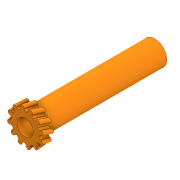
# Autodesk Inventor part: 6th Axis Drive Gear
Saved by Autodesk Inventor 2020 (Build 240168000, 168)
## iProperties
Created: 2021-06-26
Part Number: 6th Axis Drive Gear
Material: Generic
Document SubType Name: Modeling
Designer: Coy
Density: 1 g/cm^3
Appearance: Orange
Author: Coy
Autodesk Inventor part; units mm, degrees
ref_plane "YZ Plane" through (0, 0, 0) normal (1, 0, 0) x (0, 1, 0)
ref_plane "XZ Plane" through (0, 0, 0) normal (0, 1, 0) x (-1, 0, 0)
ref_plane "XY Plane" through (0, 0, 0) normal (0, 0, 1) x (1, 0, 0)
sketch "Sketch1" plane through (0, 0, 0) normal (0, 0, 1) x (1, 0, 0)
  circle A0 centre (0, 0) radius 6
  circle A1 centre (0, 0) radius 4
  dimension "d0" = 12
  dimension "d1" = 8
  constraints: 2 centre point, 2 coincident
  measures "d0" diameter of A0
  measures "d1" diameter of A1
extrude "Extrusion1" add sketch "Sketch1" along normal blind 64
ref_plane "Work Plane1" through (0, 0, 59) normal (0, 0, 1) x (1, 0, 0)
sketch "Sketch3" plane through (0, 0, 59) normal (0, 0, 1) x (1, 0, 0)
  circle A0 centre (0, 0) radius 9 construction
  line L0 (0, 0) -> (0, 12.6583) construction
  arc A1 (0.9922, 7.875) -> (-0.9922, 7.875) centre (0, 8) ccw
  line L1 (0.967, 7.675) -> (0.9922, 7.875)
  line L2 (-0.967, 7.675) -> (-0.9922, 7.875)
  arc A2 (-1.7079, 6.582) -> (-0.967, 7.675) centre (-1.9591, 7.55) ccw
  arc A3 (0.967, 7.675) -> (1.7079, 6.582) centre (1.9591, 7.55) ccw
  arc A4 (-4.7701, 4.8462) -> (-4.6749, 6.1632) centre (-5.4716, 5.5589) ccw
  line L3 (-4.6749, 6.1632) -> (-4.7967, 6.3239)
  arc A5 (-3.0783, 7.316) -> (-4.7967, 6.3239) centre (-4, 6.9282) ccw
  line L4 (-3.0001, 7.1302) -> (-3.0783, 7.316)
  arc A6 (-3.0001, 7.1302) -> (-1.8119, 6.5542) centre (-2.0783, 7.518) ccw
  arc A7 (-6.5542, 1.8119) -> (-7.1302, 3.0001) centre (-7.518, 2.0783) ccw
  line L5 (-7.1302, 3.0001) -> (-7.316, 3.0783)
  arc A8 (-6.3239, 4.7967) -> (-7.316, 3.0783) centre (-6.9282, 4) ccw
  line L6 (-6.1632, 4.6749) -> (-6.3239, 4.7967)
  arc A9 (-6.1632, 4.6749) -> (-4.8462, 4.7701) centre (-5.5589, 5.4716) ccw
  arc A10 (-6.582, -1.7079) -> (-7.675, -0.967) centre (-7.55, -1.9591) ccw
  line L7 (-7.675, -0.967) -> (-7.875, -0.9922)
  arc A11 (-7.875, 0.9922) -> (-7.875, -0.9922) centre (-8, 0) ccw
  line L8 (-7.675, 0.967) -> (-7.875, 0.9922)
  arc A12 (-7.675, 0.967) -> (-6.582, 1.7079) centre (-7.55, 1.9591) ccw
  arc A13 (-4.8462, -4.7701) -> (-6.1632, -4.6749) centre (-5.5589, -5.4716) ccw
  line L9 (-6.1632, -4.6749) -> (-6.3239, -4.7967)
  arc A14 (-7.316, -3.0783) -> (-6.3239, -4.7967) centre (-6.9282, -4) ccw
  line L10 (-7.1302, -3.0001) -> (-7.316, -3.0783)
  arc A15 (-7.1302, -3.0001) -> (-6.5542, -1.8119) centre (-7.518, -2.0783) ccw
  arc A16 (-1.8119, -6.5542) -> (-3.0001, -7.1302) centre (-2.0783, -7.518) ccw
  line L11 (-3.0001, -7.1302) -> (-3.0783, -7.316)
  arc A17 (-4.7967, -6.3239) -> (-3.0783, -7.316) centre (-4, -6.9282) ccw
  line L12 (-4.6749, -6.1632) -> (-4.7967, -6.3239)
  arc A18 (-4.6749, -6.1632) -> (-4.7701, -4.8462) centre (-5.4716, -5.5589) ccw
  arc A19 (1.7079, -6.582) -> (0.967, -7.675) centre (1.9591, -7.55) ccw
  line L13 (0.967, -7.675) -> (0.9922, -7.875)
  arc A20 (-0.9922, -7.875) -> (0.9922, -7.875) centre (0, -8) ccw
  line L14 (-0.967, -7.675) -> (-0.9922, -7.875)
  arc A21 (-0.967, -7.675) -> (-1.7079, -6.582) centre (-1.9591, -7.55) ccw
  arc A22 (4.7701, -4.8462) -> (4.6749, -6.1632) centre (5.4716, -5.5589) ccw
  line L15 (4.6749, -6.1632) -> (4.7967, -6.3239)
  arc A23 (3.0783, -7.316) -> (4.7967, -6.3239) centre (4, -6.9282) ccw
  line L16 (3.0001, -7.1302) -> (3.0783, -7.316)
  arc A24 (3.0001, -7.1302) -> (1.8119, -6.5542) centre (2.0783, -7.518) ccw
  arc A25 (6.5542, -1.8119) -> (7.1302, -3.0001) centre (7.518, -2.0783) ccw
  line L17 (7.1302, -3.0001) -> (7.316, -3.0783)
  arc A26 (6.3239, -4.7967) -> (7.316, -3.0783) centre (6.9282, -4) ccw
  line L18 (6.1632, -4.6749) -> (6.3239, -4.7967)
  arc A27 (6.1632, -4.6749) -> (4.8462, -4.7701) centre (5.5589, -5.4716) ccw
  arc A28 (6.582, 1.7079) -> (7.675, 0.967) centre (7.55, 1.9591) ccw
  line L19 (7.675, 0.967) -> (7.875, 0.9922)
  arc A29 (7.875, -0.9922) -> (7.875, 0.9922) centre (8, 0) ccw
  line L20 (7.675, -0.967) -> (7.875, -0.9922)
  arc A30 (7.675, -0.967) -> (6.582, -1.7079) centre (7.55, -1.9591) ccw
  arc A31 (4.8462, 4.7701) -> (6.1632, 4.6749) centre (5.5589, 5.4716) ccw
  line L21 (6.1632, 4.6749) -> (6.3239, 4.7967)
  arc A32 (7.316, 3.0783) -> (6.3239, 4.7967) centre (6.9282, 4) ccw
  line L22 (7.1302, 3.0001) -> (7.316, 3.0783)
  arc A33 (7.1302, 3.0001) -> (6.5542, 1.8119) centre (7.518, 2.0783) ccw
  arc A34 (1.8119, 6.5542) -> (3.0001, 7.1302) centre (2.0783, 7.518) ccw
  line L23 (3.0001, 7.1302) -> (3.0783, 7.316)
  arc A35 (4.7967, 6.3239) -> (3.0783, 7.316) centre (4, 6.9282) ccw
  line L24 (4.6749, 6.1632) -> (4.7967, 6.3239)
  arc A36 (4.6749, 6.1632) -> (4.7701, 4.8462) centre (5.4716, 5.5589) ccw
  arc A37 (-1.7079, 6.582) -> (-1.8119, 6.5542) centre (0, 0) ccw
  arc A38 (1.8119, 6.5542) -> (1.7079, 6.582) centre (0, 0) ccw
  arc A39 (4.8462, 4.7701) -> (4.7701, 4.8462) centre (0, 0) ccw
  arc A40 (6.582, 1.7079) -> (6.5542, 1.8119) centre (0, 0) ccw
  arc A41 (6.5542, -1.8119) -> (6.582, -1.7079) centre (0, 0) ccw
  arc A42 (4.7701, -4.8462) -> (4.8462, -4.7701) centre (0, 0) ccw
  arc A43 (1.7079, -6.582) -> (1.8119, -6.5542) centre (0, 0) ccw
  arc A44 (-1.8119, -6.5542) -> (-1.7079, -6.582) centre (0, 0) ccw
  arc A45 (-4.8462, -4.7701) -> (-4.7701, -4.8462) centre (0, 0) ccw
  arc A46 (-6.582, -1.7079) -> (-6.5542, -1.8119) centre (0, 0) ccw
  arc A47 (-4.7701, 4.8462) -> (-4.8462, 4.7701) centre (0, 0) ccw
  arc A48 (-6.5542, 1.8119) -> (-6.582, 1.7079) centre (0, 0) ccw
  circle A49 centre (0, 0) radius 6 projected
  dimension "d8" = 18
  dimension "d10" = 2
  dimension "d11" = 2
  dimension "d12" = 2
  dimension "d15" = 360
  constraints: 96 point on circle, 50 end point, 49 centre point, 24 line through centre, 5 tangent, 1 coincident, 1 point on line, 1 vertical, 169 other
  measures "d8" diameter of A0
  measures "d10" diameter of A1
  measures "d11" diameter of A2
  measures "d12" diameter of A3
sketch3d "3D Sketch1"
  helix H0 starts at (4.8423, -4.7663, 59) axis through (0, 0, 59) along (0, 0, 1) pitch 166.6667 turns 0.03 hand right
sweep "Sweep1" add profiles "Sketch3" path "3D Sketch1"
body "Solid1"
